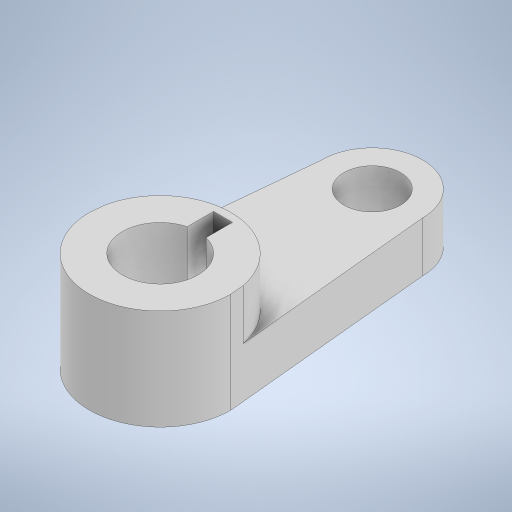
# Autodesk Inventor part: trial 3
Saved by Autodesk Inventor 2023.6 (Build 276521000, 521)
## iProperties
Created: 2026-04-03
Part Number: trial 3
Material: Generic
Document SubType Name: Modeling
Designer: ADMIN
Density: 1 g/cm^3
Appearance: Default
Author: ADMIN
Autodesk Inventor part; units mm, degrees
ref_plane "YZ Plane" through (0, 0, 0) normal (1, 0, 0) x (0, 1, 0)
ref_plane "XZ Plane" through (0, 0, 0) normal (0, 1, 0) x (-1, 0, 0)
ref_plane "XY Plane" through (0, 0, 0) normal (0, 0, 1) x (1, 0, 0)
sketch "Sketch1" plane through (0, 0, 0) normal (0, 1, 0) x (-1, 0, 0)
  circle A0 centre (52.8488, -66.0197) radius 22.5
  arc A1 (55.8488, -77.6386) -> (49.8488, -77.6386) centre (52.8488, -66.0197) ccw
  line L0 (52.8488, -88.5197) -> (52.8488, -133.5197)
  line L1 (52.8488, -88.5197) -> (97.8488, -88.5197) construction
  line L2 (52.8488, -133.5197) -> (52.8488, -149.5197)
  circle A2 centre (52.8488, -133.5197) radius 9
  line L3 (52.8488, -133.5197) -> (68.8488, -133.5197)
  line L4 (52.8488, -133.5197) -> (60.8488, -147.3761)
  line L5 (52.8488, -133.5197) -> (68.8488, -133.5197) construction
  line L6 (52.8488, -133.5197) -> (44.8488, -147.3761)
  line L7 (52.8488, -133.5197) -> (68.8488, -133.5197) construction
  line L8 (52.8488, -133.5197) -> (49.8488, -133.5197)
  arc A3 (36.8488, -133.5197) -> (68.8488, -133.5197) centre (52.8488, -133.5197) ccw
  line L9 (52.8488, -66.0197) -> (75.3488, -66.0197)
  line L10 (52.8488, -66.0197) -> (30.3488, -66.0197)
  line L11 (75.3488, -66.0197) -> (68.8488, -133.5197)
  line L12 (30.3488, -66.0197) -> (36.8488, -133.5197)
  line L13 (52.8488, -78.0197) -> (55.8488, -78.0197)
  line L14 (52.8488, -78.0197) -> (55.8488, -78.0197) construction
  line L15 (55.8488, -78.0197) -> (55.8488, -86.0197)
  line L16 (55.8488, -86.0197) -> (49.8488, -86.0197)
  line L17 (52.8488, -78.0197) -> (49.8488, -78.0197)
  line L18 (52.8488, -78.0197) -> (55.8488, -78.0197) construction
  line L19 (49.8488, -78.0197) -> (49.8488, -86.0197)
  line L20 (55.8488, -78.0197) -> (55.8488, -77.6386)
  line L21 (49.8488, -78.0197) -> (49.8488, -77.6386)
  point P0 (0, 0)
  point P1 (30.7622, -70.3132)
  point P2 (74.9353, -70.3132)
  dimension "d0" = 45
  dimension "d1" = 24
  dimension "d2" = 45
  dimension "d3" = 90
  dimension "d4" = 18
  dimension "d5" = 16
  dimension "d6" = 16
  dimension "d7" = 60
  dimension "d8" = 16
  dimension "d9" = 120
  dimension "d10" = 16
  dimension "d11" = 16
  dimension "d12" = 3
  dimension "d13" = 0
  dimension "d14" = 8
  dimension "d15" = 6
  dimension "d16" = 3
  dimension "d17" = 180
  constraints: 44 end point, 10 horizontal, 8 point on circle, 4 centre point, 3 equal length, 2 coincident, 2 perpendicular, 2 tangent, 2 vertical, 1 point on line
  measures "d0" diameter of A0
  measures "d1" diameter of A1
  measures "d2" distance of L0.start L0.end
  measures "d3" angle of L0 L1
  measures "d4" diameter of A2
  measures "d5" distance of L3.start L3.end
  measures "d6" distance of L3.start L4.end
  measures "d7" angle of L4 L5
  measures "d8" distance of L3.start L6.end
  measures "d9" angle of L6 L7
  measures "d10" distance of L3.start L12.end
  measures "d11" radius of A3
  measures "d12" distance of L13.start L13.end
  measures "d13" distance between parallel lines of L13 L14
  measures "d14" distance of L13.end L15.end
  measures "d15" distance of L15.end L16.end
  measures "d16" distance of L13.start L17.end
  measures "d17" angle of L17 L18
extrude "Extrusion1" add sketch "Sketch1" along normal blind 32 contours L9 A1 L10 A0 | L11 A0 L12 L10 A1 L21 L19 L16 L15 L20 L9
extrude "Extrusion2" add sketch "Sketch1" along normal blind 16 contours L11 L3 A2 L0 A0 | A0 L0 A2 L6 A3 L12 | A3 L4 A2 L3 | A3 L2 A2 L4 | L6 A2 L2 A3
body "Solid1"
